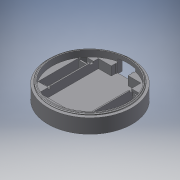
# Autodesk Inventor part: Bauteil6
Saved by Autodesk Inventor 2016 SP2 (Build 200236200, 236)
## iProperties
Created: 2018-09-27
Part Number: Bauteil6
Material: Generisch
Document SubType Name: Modeling
Designer: Nils
Density: 1 g/cm^3
Appearance: Vorgabe
Author: Nils
Autodesk Inventor part; units mm, degrees
ref_plane "YZ Plane" through (0, 0, 0) normal (1, 0, 0) x (0, 1, 0)
ref_plane "XZ Plane" through (0, 0, 0) normal (0, 1, 0) x (-1, 0, 0)
ref_plane "XY Plane" through (0, 0, 0) normal (0, 0, 1) x (1, 0, 0)
sketch "Skizze1" plane through (0, 0, 0) normal (0, 1, 0) x (-1, 0, 0)
  line L0 (0, 0) -> (-50, 0)
  line L1 (-50, 0) -> (-50, 20) construction
  line L2 (-50, 20) -> (-45, 20) construction
  line L3 (-45, 20) -> (-45, 2)
  line L4 (-45, 2) -> (0, 2)
  line L5 (-45, 20) -> (-47.3, 20)
  line L6 (-47.3, 20) -> (-47.3, 17)
  line L7 (-47.3, 17) -> (-50, 17)
  line L8 (-50, 17) -> (-50, 0)
  line L9 (0, 0) -> (0, 2)
  dimension "d0" = 50
  dimension "d1" = 20
  dimension "d2" = 5
  dimension "d3" = 2
  dimension "d4" = 2.3
  dimension "d5" = 3
  constraints: 20 end point, 4 perpendicular, 2 horizontal, 2 point on line, 2 vertical, 1 parallel
  measures "d0" distance of L0.start L0.end
  measures "d1" distance of L0.end L1.end
  measures "d2" distance of L1.end L2.end
  measures "d3" distance between parallel lines of L0 L4
  measures "d4" distance of L2.end L5.end
  measures "d5" distance of L5.end L6.end
revolve "Umdrehung1" add sketch "Skizze1" angle 360 about axis through (0, 0, 0) along (0, 0, 1)
thread "Gewinde1" size "M95x2" class "6g" standard "ANSI Metric M Profile" full length
sketch "Skizze5" plane through (0, 0, 2) normal (0, 0, 1) x (1, 0, 0)
  line L0 (-25.35, -35.35) -> (25.35, -35.35)
  line L1 (25.35, -35.35) -> (25.35, 35.35)
  line L2 (25.35, 35.35) -> (-25.35, 35.35)
  line L3 (-25.35, 35.35) -> (-25.35, -35.35)
  line L4 (-37.55, 23.95) -> (-26.55, 23.95)
  line L5 (-26.55, 23.95) -> (-26.55, -24.35)
  line L6 (-26.55, -24.35) -> (-37.55, -24.35)
  line L7 (-37.55, -24.35) -> (-37.55, 23.95)
  line L8 (26.55, 23.95) -> (37.55, 23.95)
  line L9 (37.55, 23.95) -> (37.55, -24.35)
  line L10 (37.55, -24.35) -> (26.55, -24.35)
  line L11 (26.55, -24.35) -> (26.55, 23.95)
  line L12 (-32.05, 23.95) -> (-32.1521, 39.9511) construction
  line L13 (-32.05, -24.35) -> (-31.6399, -40.3462) construction
  line L14 (32.05, 23.95) -> (32.1521, 39.9511) construction
  line L15 (32.05, -24.35) -> (31.6399, -40.3462) construction
  line L16 (-37.55, -0.2) -> (-40.85, -0.2) construction
  line L17 (37.55, -0.2) -> (40.85, -0.2) construction
  line L18 (-34.1135, -24.35) -> (-27.05, -22.35)
  line L19 (-27.05, -22.35) -> (-30.8, -20.55)
  line L20 (-30.8, -20.55) -> (-33.8, -20.55)
  line L21 (-33.8, -20.55) -> (-33.8, -21.35)
  line L22 (-33.8, -21.35) -> (-30.9821, -21.35)
  line L23 (-30.9821, -21.35) -> (-29.3023, -22.1563)
  line L24 (-29.3023, -22.1563) -> (-37.05, -24.35)
  line L25 (33.3, 20.15) -> (30.3, 20.15)
  line L26 (30.3, 20.15) -> (30.3, 20.95)
  line L27 (30.3, 20.95) -> (33.1179, 20.95)
  line L28 (37.05, 21.95) -> (29.9865, 23.95)
  line L29 (34.7977, 21.7563) -> (27.05, 23.95)
  line L30 (33.1179, 20.95) -> (34.7977, 21.7563)
  line L31 (33.3, 20.15) -> (37.05, 21.95)
  line L32 (-36.55, 25.55) -> (-27.55, 25.55)
  line L33 (-27.55, 25.55) -> (-27.55, 26.55)
  line L34 (-27.55, 26.55) -> (-36.55, 26.55) construction
  line L35 (-36.55, 26.55) -> (-36.55, 25.55)
  line L36 (36.55, -26.95) -> (27.55, -26.95) construction
  line L37 (27.55, -26.95) -> (27.55, -25.95)
  line L38 (27.55, -25.95) -> (36.55, -25.95)
  line L39 (36.55, -25.95) -> (36.55, -26.95)
  circle A0 centre (0, 0) radius 45 projected
  line L40 (27.55, -25.95) -> (27.55, -29.95)
  line L41 (27.55, -29.95) -> (33.3, -29.95)
  line L42 (33.3, -29.95) -> (36.55, -25.95)
  line L43 (-27.55, 25.55) -> (-27.55, 29.55)
  line L44 (-27.55, 29.55) -> (-33.3, 29.55)
  line L45 (-33.3, 29.55) -> (-36.55, 25.55)
  dimension "d28" = 50.7
  dimension "d29" = 70.7
  dimension "d32" = 11
  dimension "d33" = 11
  dimension "d34" = 48.3
  dimension "d35" = 48.3
  dimension "d36" = 1.2
  dimension "d37" = 1.2
  dimension "d38" = 0.8
  dimension "d39" = 0.8
  dimension "d40" = 0.8
  dimension "d41" = 3
  dimension "d42" = 3.75
  dimension "d43" = 2
  dimension "d44" = 3
  dimension "d45" = 0.5
  dimension "d46" = 0.5
  dimension "d47" = 0.8
  dimension "d48" = 0.5
  dimension "d49" = 3
  dimension "d50" = 3.75
  dimension "d51" = 2
  dimension "d52" = 0.5
  dimension "d53" = 3
  dimension "d54" = 0.8
  dimension "d55" = 0.8
  dimension "d56" = 1.6
  dimension "d57" = 1
  dimension "d58" = 1
  dimension "d59" = 1
  dimension "d60" = 1
  dimension "d61" = 1
  dimension "d62" = 1
  dimension "d63" = 1.6
  dimension "d65" = 35.35
  dimension "d66" = 25.35
  dimension "d67" = 8.4
  dimension "d68" = 11
  dimension "d108" = 4
  dimension "d109" = 4
  dimension "d110" = 5.75
  dimension "d111" = 5.75
  constraints: 92 end point, 15 parallel, 11 perpendicular, 6 horizontal, 6 midpoint, 6 point on line, 3 equal length, 2 vertical
  measures "d28" distance of L2.end L1.end
  measures "d29" distance of L1.end L0.end
  measures "d32" distance between parallel lines of L5 L7
  measures "d33" distance of L8.start L8.end
  measures "d34" distance between parallel lines of L6 L4
  measures "d35" distance of L8.end L9.end
  measures "d36" distance between parallel lines of L3 L5
  measures "d37" distance between parallel lines of L11 L1
  measures "d38" distance between parallel lines of L18 L24
  measures "d39" distance between parallel lines of L19 L23
  measures "d40" distance between parallel lines of L22 L20
  measures "d41" distance of L19.end L20.end
  measures "d42" distance between parallel lines of L7 L21
  measures "d43" distance from line of L6 L18.end
  measures "d44" distance between parallel lines of L6 L22
  measures "d45" distance of L24.end L6.end
  measures "d46" distance from line of L5 L18.end
  measures "d47" distance between parallel lines of L25 L27
  measures "d48" distance from line of L9 L28.start
  measures "d49" distance of L25.start L25.end
  measures "d50" distance between parallel lines of L11 L26
  measures "d51" distance from line of L8 L28.start
  measures "d52" distance of L8.start L29.end
  measures "d53" distance between parallel lines of L8 L27
  measures "d54" distance between parallel lines of L31 L30
  measures "d55" distance between parallel lines of L28 L29
  measures "d56" distance between parallel lines of L4 L32
  measures "d57" distance between parallel lines of L35 L7
  measures "d58" distance between parallel lines of L5 L33
  measures "d59" distance between parallel lines of L32 L34
  measures "d60" distance of L36.end L37.end
  measures "d61" distance between parallel lines of L9 L39
  measures "d62" distance between parallel lines of L37 L11
  measures "d63" distance between parallel lines of L38 L10
  measures "d65" distance from line of point (0, 0) L0
  measures "d66" distance from line of point (0, 0) L3
  measures "d67" distance between parallel lines of L36 L0
  measures "d68" distance between parallel lines of L0 L6
  measures "d108" distance of L37.end L40.end
  measures "d109" distance of L32.end L43.end
  measures "d110" distance of L43.end L44.end
  measures "d111" distance of L40.end L41.end
extrude "Extrusion1" add sketch "Skizze5" along normal blind 10.5 contours L24 L23 L22 L21 L20 L19 L18 L6 | L8 L28 L31 L25 L26 L27 L30 L29 | A0
sketch "Skizze6" plane through (-33.8, -20.55, 2) normal (0, 1, 0) x (1, 0, 0)
  line L0 (7.25, 0) -> (7.25, -10.5) projected
  line L1 (-3.75, 0) -> (-3.75, -10.5) projected
  line L2 (7.25, 0) -> (-3.75, 0)
  line L3 (-3.75, 0) -> (-3.75, -3)
  line L4 (-3.75, -3) -> (7.25, -3)
  line L5 (7.25, -3) -> (7.25, 0)
  line L6 (-3.75, -10.5) -> (7.25, -10.5)
  line L7 (7.25, -10.5) -> (7.25, -7.5)
  line L8 (7.25, -7.5) -> (-3.75, -7.5)
  line L9 (-3.75, -7.5) -> (-3.75, -10.5)
  point P0 (33.8, 2)
  dimension "d71" = 3
  dimension "d72" = 3
  constraints: 16 end point, 4 parallel, 2 horizontal, 2 perpendicular, 2 point on line
  measures "d71" distance of L3.end L2.end
  measures "d72" distance of L7.end L6.end
extrude "Extrusion2" cut sketch "Skizze6" against normal blind 3.8 contours L0 L4 L1 L2 | L0 L6 L1 L8
sketch "Skizze7" plane through (30.3, 20.15, 2) normal (0, -1, 0) x (1, 0, 0)
  line L0 (7.25, 0) -> (7.25, 10.5) projected
  line L1 (-3.75, 0) -> (-3.75, 10.5) projected
  line L2 (-3.75, 0) -> (7.25, 0)
  line L3 (7.25, 0) -> (7.25, 3)
  line L4 (7.25, 3) -> (-3.75, 3)
  line L5 (-3.75, 3) -> (-3.75, 0)
  line L6 (7.25, 10.5) -> (-3.75, 10.5)
  line L7 (-3.75, 10.5) -> (-3.75, 7.5)
  line L8 (-3.75, 7.5) -> (7.25, 7.5)
  line L9 (7.25, 7.5) -> (7.25, 10.5)
  point P0 (-30.3, -2)
  dimension "d75" = 3
  dimension "d76" = 3
  constraints: 16 end point, 4 parallel, 2 horizontal, 2 perpendicular, 2 point on line
  measures "d75" distance of L3.end L2.end
  measures "d76" distance of L7.end L6.end
extrude "Extrusion3" cut sketch "Skizze7" against normal blind 3.8 contours L2 L1 L4 L0 | L8 L1 L6 L0
thread "Gewinde2" size "M95x2" class "6g" standard "ANSI Metric M Profile" full length
sketch "Skizze9" plane through (0, 0, 20) normal (-1, 0, 0) x (0, 1, 0)
  line L0 (47.3, 0) -> (47.3, 3)
  line L1 (47.3, 3) -> (45.9948, 3)
  line L2 (45.9948, 3) -> (45.9948, 0)
  line L3 (45.9948, 0) -> (47.3, 0)
  line L4 (0, -4.15) -> (0, 24.9) projected
  constraints: 8 end point
revolve "Umdrehung4" cut sketch "Skizze9" angle 360 about axis through (0, 0, 20) along (0, 0, -1)
sketch "Skizze10" plane through (0, 0, 20) normal (-1, 0, 0) x (0, 1, 0)
  line L0 (47.3, 0) -> (47.3, 3)
  line L1 (47.3, 3) -> (45.9948, 3)
  line L2 (45.9948, 3) -> (45.9948, 0)
  line L3 (45.9948, 0) -> (47.3, 0)
  line L4 (0, -4.15) -> (0, 24.9) projected
  constraints: 8 end point
revolve "Umdrehung5" add sketch "Skizze10" angle 360 about axis through (0, 0, 20) along (0, 0, -1) separate body
sketch "Skizze8" plane through (0, 0, 20) normal (1, 0, 0) x (0, 0, -1)
  line L0 (-1.1849, -46.1017) -> (-1.0001, -46.1017) construction
  line L1 (0.1847, -47.1934) -> (-0.0001, -47.5136) construction
  line L2 (-2.0001, -47.5136) -> (-2.185, -47.1934) construction
  line L3 (-0.8153, -46.1017) -> (-1.0001, -45.7816) construction
  line L4 (-1.0001, -45.7816) -> (-1.1849, -46.1017) construction
  line L5 (-2.0001, -47.5136) -> (-1.8153, -47.1934) construction
  line L6 (-0.8153, -46.1017) -> (-0.1849, -47.1934)
  line L7 (-2.185, -47.1934) -> (-1.8153, -47.1934) construction
  arc A0 (-2.185, -47.1934) -> (-2.0001, -47.3002) centre (-2.0001, -47.0867) ccw construction
  line L8 (0.1847, -47.1934) -> (-0.1849, -47.1934) construction
  line L9 (-2.0001, -47.5136) -> (-2.0001, -47.1934) construction
  line L10 (-0.0001, -47.5136) -> (-0.0001, -47.1934) construction
  line L11 (-1.0001, -45.7816) -> (-1.0001, -45.995) construction
  line L12 (-2.0001, -47.3002) -> (-0.0001, -47.3002)
  arc A1 (-2.0001, -47.3002) -> (-1.8153, -47.1934) centre (-2.0001, -47.0867) ccw
  line L13 (-0.1849, -47.1934) -> (-0.0001, -47.5136) construction
  line L14 (-1.8153, -47.1934) -> (-1.1849, -46.1017)
  line L15 (-0.0001, -0.0002) -> (-0.0001, 0.0177)
  line L16 (-0.0001, 0.0177) -> (-0.0001, -0.0002)
  line L17 (-0.0001, -0.0002) -> (0.0334, -0.0002)
  arc A2 (-0.1849, -47.1934) -> (-0.0001, -47.3002) centre (-0.0001, -47.0867) ccw
  arc A3 (-0.0001, -47.3002) -> (0.1847, -47.1934) centre (-0.0001, -47.0867) ccw construction
  arc A4 (-1.0001, -45.995) -> (-1.1849, -46.1017) centre (-1.0001, -46.2084) ccw
  arc A5 (-0.8153, -46.1017) -> (-1.0001, -45.995) centre (-1.0001, -46.2084) ccw
  line L18 (-1.0001, -45.995) -> (-1.0001, -46.1017) construction
  line L19 (-1.0001, -46.1017) -> (-0.8153, -46.1017) construction
  dimension "d81" = 60
  dimension "d82" = 0.3202
  dimension "d83" = 0.3202
  dimension "Skizze8_ThreadOffset" = 0
  dimension "Skizze8_MajorRadius" = 47.3
  dimension "d86" = 2
  dimension "Skizze8_MinorRadius" = 45.9948
  constraints: 40 end point, 12 point on circle, 10 parallel, 8 tangent, 6 centre point, 6 collinear, 2 midpoint, 2 point on line, 1 horizontal, 1 perpendicular, 3 other
  measures "d81" angle of L6 L14
  measures "d82" distance of L3.end L0.end
  measures "d83" distance of L1.end L10.end
  measures "Skizze8_ThreadOffset" distance between parallel lines of L15 L10
  measures "Skizze8_MajorRadius" distance from line of L12 L15.start
  measures "d86" distance from line of L1.end L9
  measures "Skizze8_MinorRadius" distance edge to line of A5 L17
coil "Spirale2" sketch "Skizze8" operation cut axis through (0, 0, 20) along (0, 0, -1) pitch 2.002 turns 3.496503 hand right bodies 2
sketch "Skizze11" plane through (-25.35, 35.35, 2) normal (0, -1, 0) x (1, 0, 0)
  line L0 (34.85, 0) -> (15.85, 0)
  line L1 (15.85, 0) -> (15.85, 11.5)
  line L2 (15.85, 11.5) -> (34.85, 11.5)
  line L3 (34.85, 11.5) -> (34.85, 0)
  line L4 (50.7, 0) -> (0, 0) projected
  line L5 (15.85, 5.75) -> (0, 5.75) construction
  line L6 (0, 0) -> (0, 10.5) construction
  line L7 (34.85, 5.75) -> (50.7, 5.75) construction
  line L8 (50.7, 0) -> (50.7, 10.5) construction
  point P0 (25.35, -2)
  dimension "d100" = 19
  dimension "d101" = 11.5
  constraints: 12 end point, 3 point on line, 2 collinear, 2 horizontal, 2 midpoint, 2 parallel, 1 perpendicular
  measures "d100" distance of L1.end L2.end
  measures "d101" distance of L0.end L1.end
extrude "Extrusion4" cut sketch "Skizze11" against normal blind 7 bodies 1
sketch "Skizze12" plane through (-25.35, 42.35, 2) normal (0, -1, 0) x (1, 0, 0)
  line L0 (34.85, 0) -> (15.85, 0) construction
  line L1 (25.35, 0) -> (25.35, 11.5) construction
  line L2 (16.35, 11.5) -> (34.35, 11.5) construction
  line L3 (14.85, -2) -> (35.85, -2)
  line L4 (35.85, -2) -> (35.85, 13.5)
  line L5 (35.85, 13.5) -> (14.85, 13.5)
  line L6 (14.85, 13.5) -> (14.85, -2)
  line L7 (14.85, -2) -> (35.85, 13.5) construction
  line L8 (35.85, -2) -> (14.85, 13.5) construction
  point P0 (25.35, -2)
  point P1 (25.35, 5.75)
  dimension "d104" = 21
  dimension "d105" = 15.5
  constraints: 14 end point, 5 midpoint, 2 parallel, 1 horizontal, 1 perpendicular
  measures "d104" distance of L5.end L4.end
  measures "d105" distance of L4.end L3.end
extrude "Extrusion5" cut sketch "Skizze12" against normal blind 9.5 bodies 1
sketch "Skizze13" plane through (0, 0, 12.5) normal (0, 0, 1) x (1, 0, 0)
  line L0 (-25.35, -35.35) -> (-25.35, 35.35) projected
  line L1 (-27.55, 29.55) -> (-27.55, 25.55) projected
  line L2 (-25.35, 29.55) -> (-27.55, 29.55)
  line L3 (-27.55, 29.55) -> (-27.55, 25.55)
  line L4 (-27.55, 25.55) -> (-25.35, 25.55)
  line L5 (-25.35, 25.55) -> (-25.35, 29.55)
  line L6 (25.35, -35.35) -> (25.35, 35.35) projected
  line L7 (27.55, -29.95) -> (27.55, -25.95) projected
  line L8 (25.35, -29.95) -> (27.55, -29.95)
  line L9 (27.55, -29.95) -> (27.55, -25.95)
  line L10 (27.55, -25.95) -> (25.35, -25.95)
  line L11 (25.35, -25.95) -> (25.35, -29.95)
  line L12 (26.55, 23.95) -> (26.55, -24.35) projected
  line L13 (26.55, 23.95) -> (25.35, 23.95)
  line L14 (25.35, 23.95) -> (25.35, 20.95)
  line L15 (25.35, 20.95) -> (26.55, 20.95)
  line L16 (26.55, 20.95) -> (26.55, 23.95)
  line L17 (-26.55, 23.95) -> (-26.55, -24.35) projected
  line L18 (-26.55, -24.35) -> (-25.35, -24.35)
  line L19 (-25.35, -24.35) -> (-25.35, -21.35)
  line L20 (-25.35, -21.35) -> (-26.55, -21.35)
  line L21 (-26.55, -21.35) -> (-26.55, -24.35)
  line L22 (-37.55, 23.95) -> (-26.55, 23.95) projected
  line L23 (-36.55, 25.55) -> (-27.75, 25.55)
  line L24 (-27.75, 25.55) -> (-27.75, 23.95)
  line L25 (-27.75, 23.95) -> (-36.55, 23.95)
  line L26 (-36.55, 23.95) -> (-36.55, 25.55)
  line L27 (37.55, -24.35) -> (26.55, -24.35) projected
  line L28 (36.6361, -25.95) -> (27.75, -25.95)
  line L29 (27.75, -25.95) -> (27.75, -24.35)
  line L30 (27.75, -24.35) -> (36.6361, -24.35)
  line L31 (36.6361, -24.35) -> (36.6361, -25.95)
  point P0 (0, 0)
  dimension "d112" = 3
  dimension "d113" = 3
  dimension "d114" = 4
  dimension "d115" = 4
  constraints: 48 end point, 12 parallel, 6 horizontal, 6 perpendicular, 6 point on line
  measures "d112" distance of L14.end L13.end
  measures "d113" distance of L19.end L18.end
  measures "d114" distance between parallel lines of L2 L4
  measures "d115" distance between parallel lines of L8 L10
extrude "Extrusion6" cut sketch "Skizze13" against normal blind 2 bodies 1
sketch "Skizze14" plane through (-25.35, 35.35, 2) normal (0, -1, 0) x (1, 0, 0)
  line L0 (15.85, 0) -> (15.85, 10.5) construction
  line L1 (15.85, 5.25) -> (34.85, 5.25) construction
  line L2 (34.85, 10.5) -> (34.85, 0) construction
  line L3 (50.7, 0) -> (34.85, 0) projected
  line L4 (15.35, 10.5) -> (35.35, 10.5)
  line L5 (35.35, 10.5) -> (35.35, 0)
  line L6 (35.35, 0) -> (15.35, 0)
  line L7 (15.35, 0) -> (15.35, 10.5)
  line L8 (15.35, 10.5) -> (35.35, 0) construction
  line L9 (35.35, 10.5) -> (15.35, 0) construction
  point P0 (25.35, -2)
  point P1 (25.35, 5.25)
  dimension "d118" = 20
  constraints: 14 end point, 5 midpoint, 2 parallel, 1 horizontal, 1 perpendicular, 1 point on line
  measures "d118" distance of L5.end L6.end
extrude "Extrusion7" cut sketch "Skizze14" against normal blind 5 bodies 1
equation "\"d33\" = d32"
equation "\"d35\" = d34"
equation "\"d48\" = d64"
equation "\"d58\" = d57"
equation "\"d62\" = d61"
equation "\"d65\" = 0.5 * d29"
equation "\"d66\" = 0.5 * d28"
equation "\"d81\" = d88"
equation "\"d82\" = 0.160083 * Skizze8_Pitch"
equation "\"d83\" = 0.160083 * Skizze8_Pitch"
equation "\"d86\" = Skizze8_Pitch"
equation "\"d16\" = 60deg"
equation "\"Skizze2_Pitch\" = 2"
equation "\"d88\" = 60deg"
equation "\"Skizze8_Pitch\" = 2"
equation "\"d64\" = 0.5"
